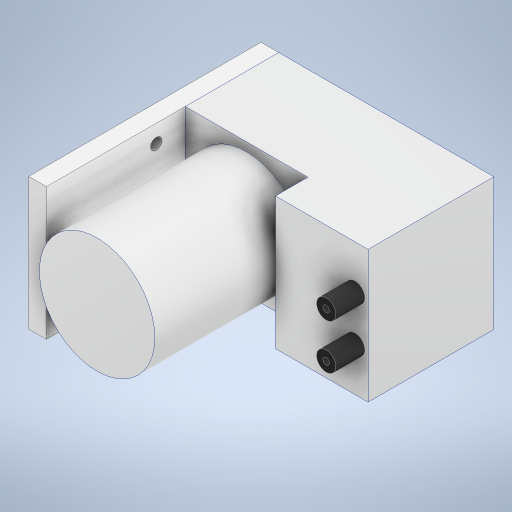
# Autodesk Inventor part: DP0110-Y1
Saved by Autodesk Inventor 2024.1 (Build 281209000, 209)
## iProperties
Created: 2023-12-30
Part Number: DP0110-Y1
Material: アルミニウム 6061
Document SubType Name: Modeling
Designer: haruy
Density: 2.7 g/cm^3
Appearance: アルミニウム - フラット
Author: haruy
Autodesk Inventor part; units mm, degrees
ref_plane "YZ Plane" through (0, 0, 0) normal (1, 0, 0) x (0, 1, 0)
ref_plane "XZ Plane" through (0, 0, 0) normal (0, 1, 0) x (-1, 0, 0)
ref_plane "XY Plane" through (0, 0, 0) normal (0, 0, 1) x (1, 0, 0)
sketch "スケッチ1" plane through (0, 0, 0) normal (1, 0, 0) x (0, 1, 0)
  line L0 (0, 0) -> (41, 0)
  line L1 (41, 0) -> (41, -39)
  line L2 (41, -39) -> (0, -39)
  line L3 (0, -39) -> (0, 0)
  dimension "d0" = 41
  dimension "d1" = 39
  constraints: 8 end point, 2 parallel, 1 horizontal, 1 perpendicular
  measures "d0" distance of L1.end L2.end
  measures "d1" distance of L0.end L1.end
extrude "押し出し1" add sketch "スケッチ1" along normal blind 66.7
sketch "スケッチ2" plane through (0, 0, -39) normal (0, -1, 0) x (1, 0, 0)
  line L0 (0, 39) -> (38, 39)
  line L1 (38, 39) -> (38, 29)
  line L2 (38, 29) -> (0, 29)
  line L3 (0, 29) -> (0, 39)
  dimension "d4" = 38
  dimension "d5" = 10
  constraints: 8 end point, 2 parallel, 1 horizontal, 1 perpendicular
  measures "d4" distance of L1.end L2.end
  measures "d5" distance of L0.end L1.end
extrude "押し出し2" cut sketch "スケッチ2" against normal through all
sketch "スケッチ3" plane through (0, 0, -10) normal (0, 0, 1) x (1, 0, 0)
  line L0 (0, 0) -> (0, 41) projected
  line L1 (38, 0) -> (0, 0) projected
  circle A0 centre (19, 20.5) radius 17.9
  dimension "d22" = 0
  dimension "d8" = 19
  dimension "d9" = 20.5
  dimension "d10" = 35.8
  constraints: 1 centre point, 1 coincident
  measures "d8" distance from line of point (19, 20.5) L0
  measures "d9" distance from line of L1 point (19, 20.5)
  measures "d10" diameter of A0
extrude "押し出し3" add sketch "スケッチ3" along normal blind 46.3
sketch "スケッチ4" plane through (0, 0, 0) normal (-1, 0, 0) x (0, 0, 1)
  circle A0 centre (-1, 5.5) radius 1.75
  circle A1 centre (-1, 35.5) radius 1.75
  line L0 (-39, 0) -> (-39, 41) projected
  line L1 (-39, 0) -> (33, 0)
  line L2 (33, 0) -> (33, 41)
  line L3 (33, 41) -> (-39, 41)
  line L4 (-39, 41) -> (-39, 0)
  point P0 (0, 0)
  dimension "d13" = 3.5
  dimension "d14" = 3.5
  dimension "d15" = 30
  dimension "d16" = 5.5
  dimension "d17" = 0
  dimension "d18" = 38
  dimension "d19" = 41
  dimension "d20" = 72
  constraints: 8 end point, 2 centre point, 2 parallel, 1 horizontal, 1 perpendicular
  measures "d13" diameter of A0
  measures "d14" diameter of A1
  measures "d15" distance of A1.centre A0.centre
  measures "d16" vertical distance of A0.centre point (0, 0)
  measures "d17" horizontal distance of A1.centre A0.centre
  measures "d18" distance from line of A0.centre L0
  measures "d19" distance of L1.end L2.end
  measures "d20" distance of L2.end L3.end
extrude "押し出し4" add sketch "スケッチ4" along normal blind 5.5 separate body
sketch "スケッチ5" plane through (66.7, 0, 0) normal (0, 0, 1) x (1, 0, 0)
  circle A0 centre (-4, 27.5) radius 3
  circle A1 centre (-4, 13.5) radius 3
  line L0 (-72.2, 0) -> (-72.2, 41) projected
  line L1 (-28.7, 41) -> (0, 41) projected
  circle A2 centre (-4, 27.5) radius 1
  circle A3 centre (-4, 13.5) radius 1
  point P0 (-66.7, 0)
  dimension "d23" = 6
  dimension "d24" = 6
  dimension "d25" = 68.2
  dimension "d26" = 68.2
  dimension "d27" = 14
  dimension "d28" = 13.5
  dimension "d29" = 2
  dimension "d30" = 2
  constraints: 4 centre point, 2 coincident
  measures "d23" diameter of A0
  measures "d24" diameter of A1
  measures "d25" distance from line of L0 A0.centre
  measures "d26" distance from line of L0 A1.centre
  measures "d27" distance of A1.centre A0.centre
  measures "d28" distance from line of A0.centre L1
  measures "d29" diameter of A2
  measures "d30" diameter of A3
extrude "押し出し5" add sketch "スケッチ5" along normal blind 9 separate body
equation "\"d26\" = d25"
